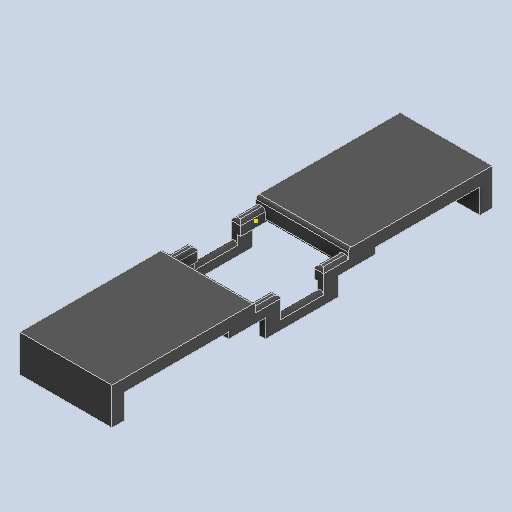
# Autodesk Inventor part: Landing dock V2
Saved by Autodesk Inventor 2023 (Build 270158000, 158)
## iProperties
Created: 2022-12-03
Part Number: Landing dock V2
Material: PLA Plastic
Document SubType Name: Modeling
Designer: cheng
Density: 1.25002 g/cm^3
Appearance: Generic
Mass: 2349.49 g
Surface Area: 2310.02 cm^2
Volume: 1879.56 cm^3
Author: cheng
Autodesk Inventor part; units mm, degrees
ref_plane "YZ Plane" through (0, 0, 0) normal (1, 0, 0) x (0, 1, 0)
ref_plane "XZ Plane" through (0, 0, 0) normal (0, 1, 0) x (-1, 0, 0)
ref_plane "XY Plane" through (0, 0, 0) normal (0, 0, 1) x (1, 0, 0)
sketch "Sketch1" plane through (0, 0, 0) normal (0, 1, 0) x (-1, 0, 0)
  line L0 (75, -309.5) -> (-75, -309.5)
  line L1 (-75, -309.5) -> (-75, 309.5)
  line L2 (-75, 309.5) -> (75, 309.5)
  line L3 (75, 309.5) -> (75, -309.5)
  line L4 (75, -309.5) -> (-75, 309.5) construction
  line L5 (-75, -309.5) -> (75, 309.5) construction
  point P0 (0, 0)
  dimension "d0" = 619
  dimension "d1" = 150
  constraints: 12 end point, 2 midpoint, 2 parallel, 1 horizontal, 1 perpendicular
  measures "d0" distance between parallel lines of L0 L2
  measures "d1" distance of L0.start L0.end
extrude "Extrusion1" add sketch "Sketch1" along normal blind 100
sketch "Sketch2" plane through (0, 100, 0) normal (0, 1, 0) x (1, 0, 0)
  point P0 (0, 0)
sketch "Sketch3" plane through (0, 100, 0) normal (0, 1, 0) x (1, 0, 0)
  line L0 (-75, -309.5) -> (75, -309.5) projected
  line L1 (75, -309.5) -> (75, 309.5) projected
  line L2 (75, 309.5) -> (-75, 309.5) projected
  line L3 (-75, 309.5) -> (-75, -309.5) projected
  line L4 (75, 309.5) -> (-75, -309.5) construction
  line L5 (-75, 309.5) -> (75, -309.5) construction
  line L6 (75, 0) -> (-75, 0) construction
  line L7 (75, 75) -> (-75, 75)
  line L8 (-75, 75) -> (-75, -75)
  line L9 (-75, -75) -> (75, -75)
  line L10 (75, -75) -> (75, 75)
  line L11 (75, 75) -> (-75, -75) construction
  line L12 (-75, 75) -> (75, -75) construction
  line L13 (0, 0) -> (75, 0) construction
  dimension "d9" = 150
  constraints: 20 end point, 4 midpoint, 2 parallel, 2 point on line, 1 collinear, 1 horizontal, 1 perpendicular
  measures "d9" distance between parallel lines of L9 L7
extrude "Extrusion2" cut sketch "Sketch3" against normal blind 50 contours L3 L7 L1 L9
sketch "Sketch5" plane through (0, 50, 0) normal (0, 1, 0) x (1, 0, 0)
  line L0 (75, 75) -> (75, -75) projected
  line L1 (-75, 75) -> (75, 75) projected
  line L2 (-75, -75) -> (-75, 75) projected
  line L3 (75, -75) -> (-75, -75) projected
  line L4 (60, 75) -> (-60, 75)
  line L5 (-60, 75) -> (-60, -75)
  line L6 (-60, -75) -> (60, -75)
  line L7 (60, -75) -> (60, 75)
  line L8 (75, 75) -> (-75, -75) construction
  line L9 (-75, 75) -> (75, -75) construction
  line L10 (75, -309.5) -> (75, 309.5) construction
  line L11 (75, 0) -> (-75, 0) construction
  line L12 (60, 75) -> (-60, -75) construction
  line L13 (-60, 75) -> (60, -75) construction
  line L14 (0, 0) -> (0, 75) construction
  line L15 (0, 0) -> (0, 75) construction
  dimension "d12" = 120
  constraints: 22 end point, 5 midpoint, 3 perpendicular, 2 parallel, 2 point on line, 1 collinear, 1 horizontal
  measures "d12" distance between parallel lines of L5 L7
extrude "Extrusion3" cut sketch "Sketch5" against normal through all contours L7 L3 L5 L1
sketch "Sketch6" plane through (0, 100, 0) normal (0, 1, 0) x (1, 0, 0)
  line L0 (75, -75) -> (-75, -75) projected
  line L1 (-75, -75) -> (-75, -309.5) projected
  line L2 (-75, -309.5) -> (75, -309.5) projected
  line L3 (75, -309.5) -> (75, -75) projected
  line L4 (-75, 75) -> (75, 75) projected
  line L5 (75, 75) -> (75, 309.5) projected
  line L6 (75, 309.5) -> (-75, 309.5) projected
  line L7 (-75, 309.5) -> (-75, 75) projected
  line L8 (-75, 309.5) -> (-75, -309.5) projected
  line L9 (-75, -309.5) -> (75, -309.5)
  line L10 (75, -309.5) -> (75, -75)
  line L11 (75, -75) -> (-75, -75)
  line L12 (-75, -75) -> (-75, -309.5)
  line L13 (-75, 75) -> (69.6165, 75)
  line L14 (69.6165, 75) -> (69.6165, 309.5)
  line L15 (69.6165, 309.5) -> (-75, 309.5)
  line L16 (-75, 309.5) -> (-75, 75)
  point P0 (0, 0)
  constraints: 16 end point, 4 parallel, 2 horizontal, 2 perpendicular, 1 point on line
extrude "Extrusion4" cut sketch "Sketch6" against normal blind 40
sketch "Sketch7" plane through (75, 0, 309.5) normal (1, 0, 0) x (0, 0, -1)
  line L0 (619, 60) -> (384.5, 60) projected
  line L1 (384.5, 60) -> (384.5, 50) projected
  line L2 (384.5, 50) -> (234.5, 50) projected
  line L3 (234.5, 50) -> (234.5, 60) projected
  line L4 (234.5, 60) -> (0, 60) projected
  line L5 (0, 0) -> (0, 60) projected
  line L6 (0, 0) -> (619, 0) projected
  line L7 (619, 0) -> (619, 60) projected
  line L8 (309.5, 0) -> (309.5, 50) construction
  line L9 (619, 0) -> (0, 0) projected
  line L10 (20, 40) -> (190, 40)
  line L11 (190, 40) -> (190, 0)
  line L12 (190, 0) -> (20, 0)
  line L13 (20, 0) -> (20, 40)
  line L14 (384.5, 50) -> (384.5, 60)
  line L15 (384.5, 60) -> (619, 60)
  line L16 (619, 0) -> (619, 60)
  line L17 (599, 40) -> (429, 40)
  line L18 (429, 40) -> (429, 0)
  line L19 (429, 0) -> (599, 0)
  line L20 (599, 0) -> (599, 40)
  point P0 (429, 0)
  dimension "d17" = 20
  dimension "d18" = 20
  dimension "d19" = 170
  constraints: 24 end point, 4 symmetric about line, 2 parallel, 1 horizontal, 1 midpoint, 1 perpendicular, 1 point on line
  measures "d17" distance between parallel lines of L10 L4
  measures "d18" distance between parallel lines of L5 L13
  measures "d19" distance between parallel lines of L13 L11
extrude "Extrusion5" cut sketch "Sketch7" against normal through all contours L6 L18 L17 L20 | L6 L13 L10 L11
sketch "Sketch8" plane through (75, 0, 119.5) normal (0, 0, 1) x (1, 0, 0)
  line L0 (-150, 0) -> (-150, 40) projected
  line L1 (0, 0) -> (-150, 0) projected
  line L2 (0, 40) -> (0, 0) projected
  line L3 (0, 40) -> (-150, 40) projected
  line L4 (-140, 0) -> (-10, 0)
  line L5 (-10, 0) -> (-10, 30)
  line L6 (-10, 30) -> (-140, 30)
  line L7 (-140, 30) -> (-140, 0)
  point P0 (-75, 0)
  dimension "d22" = 10
  dimension "d23" = 10
  dimension "d24" = 10
  constraints: 8 end point, 2 parallel, 1 horizontal, 1 perpendicular, 1 point on line
  measures "d22" distance between parallel lines of L0 L7
  measures "d23" distance between parallel lines of L2 L5
  measures "d24" distance between parallel lines of L6 L3
extrude "Extrusion6" cut sketch "Sketch8" against normal up to surface (239 mm away) contours L7 L6 L5 L1
sketch "Sketch9" plane through (75, 50, 75) normal (1, 0, 0) x (0, 0, -1)
  line L0 (364.5, -10) -> (364.5, -50) projected
  line L1 (364.5, -50) -> (384.5, -50) projected
  line L2 (384.5, -50) -> (384.5, 10) projected
  line L3 (384.5, 10) -> (150, 10) projected
  line L4 (150, 10) -> (150, 0) projected
  line L5 (150, 0) -> (0, 0) projected
  line L6 (0, 0) -> (0, 10) projected
  line L7 (0, 10) -> (-234.5, 10) projected
  line L8 (-234.5, -50) -> (-234.5, 10) projected
  line L9 (-234.5, -50) -> (-214.5, -50) projected
  line L10 (-214.5, -50) -> (-214.5, -10) projected
  line L11 (-214.5, -10) -> (-44.5, -10) projected
  line L12 (-44.5, -10) -> (-44.5, -50) projected
  line L13 (-44.5, -50) -> (194.5, -50) projected
  line L14 (194.5, -50) -> (194.5, -10) projected
  line L15 (194.5, -10) -> (364.5, -10) projected
  line L16 (75, -50) -> (75, 0) construction
  line L17 (0, 0) -> (150, 0) construction
  line L18 (40, 0) -> (110, 0)
  line L19 (110, 0) -> (110, -30)
  line L20 (110, -30) -> (40, -30)
  line L21 (40, -30) -> (40, 0)
  line L22 (40, 0) -> (110, -30) construction
  line L23 (40, -30) -> (110, 0) construction
  line L24 (75, -15) -> (75, 0) construction
  point P0 (110, 0)
  dimension "d27" = 70
  dimension "d28" = 30
  constraints: 16 end point, 3 midpoint, 2 parallel, 1 collinear, 1 horizontal, 1 perpendicular, 1 point on line
  measures "d27" distance of L19.end L20.end
  measures "d28" distance of L20.end L18.start
extrude "Extrusion7" cut sketch "Sketch9" against normal through all contours L19 L20 L21 L5
sketch "Sketch10" plane through (75, 0, 309.5) normal (1, 0, 0) x (0, 0, -1)
  line L0 (344.5, 50) -> (344.5, 20) projected
  line L1 (344.5, 20) -> (274.5, 20) projected
  line L2 (274.5, 20) -> (274.5, 50) projected
  line L3 (274.5, 50) -> (234.5, 50) projected
  line L4 (234.5, 50) -> (234.5, 60) projected
  line L5 (234.5, 60) -> (0, 60) projected
  line L6 (0, 0) -> (0, 60) projected
  line L7 (0, 0) -> (20, 0) projected
  line L8 (20, 0) -> (20, 40) projected
  line L9 (20, 40) -> (190, 40) projected
  line L10 (190, 40) -> (190, 0) projected
  line L11 (190, 0) -> (429, 0) projected
  line L12 (429, 0) -> (429, 40) projected
  line L13 (429, 40) -> (599, 40) projected
  line L14 (599, 40) -> (599, 0) projected
  line L15 (599, 0) -> (619, 0) projected
  line L16 (619, 0) -> (619, 60) projected
  line L17 (619, 60) -> (384.5, 60) projected
  line L18 (384.5, 60) -> (384.5, 50) projected
  line L19 (384.5, 50) -> (344.5, 50) projected
  line L20 (309.5, 0) -> (309.5, 20) construction
  line L21 (190, 0) -> (250, 0)
  line L22 (250, 0) -> (250, 30)
  line L23 (250, 30) -> (190, 30)
  line L24 (190, 30) -> (190, 0)
  line L25 (429, 0) -> (369, 0)
  line L26 (369, 0) -> (369, 30)
  line L27 (369, 30) -> (429, 30)
  line L28 (429, 30) -> (429, 0)
  dimension "d31" = 60
  dimension "d32" = 30
  constraints: 18 end point, 3 symmetric about line, 2 parallel, 1 horizontal, 1 midpoint, 1 perpendicular
  measures "d31" distance of L22.end L23.end
  measures "d32" distance of L21.end L22.end
extrude "Extrusion8" cut sketch "Sketch10" against normal through all contours L12 L11 L26 L27 | L23 L22 L11 L10
fillet "Fillet1" radius 5 20 edges at (-60, 50, 55) (-65, 20, 0) (-60, 50, -55) (65, 20, 0) (60, 50, 55) (75, 50, 55) (60, 50, -55) (75, 50, -55) (75, 20, 0) (-75, 20, 0) (-75, 50, 55) (-75, 50, -55) (-67.5, 50, -35) (-67.5, 50, 35) (67.5, 50, 35) (67.5, 50, -35) (0, 60, 75) (0, 60, -75) (0, 30, 75) (0, 30, -75)
body "Solid1"
